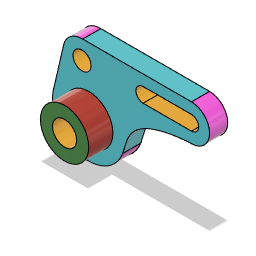
Questão4 (Autodesk Fusion 360 design; units mm, degrees)
Autodesk Fusion 360 part; units mm, degrees
sketch "Esboço1" plane through (0, 0, 0) normal (0, 0, 1) x (1, 0, 0)
  circle A0 centre (-75.5675, 24.3524) radius 7.5
  line L0 (-74.9976, 40) -> (15, 40)
  circle A1 centre (-70, -15) radius 10
  circle A2 centre (-70, -15) radius 20
  arc A3 (-74.9976, 40) -> (-91, 27) centre (-75.5675, 24.3524) ccw
  arc A4 (-98.6911, -6.2353) -> (-41.8777, -25.4469) centre (-70, -15) ccw
  line L1 (-91, 27) -> (-99.6247, -10.2696)
  spline S0 degree 5 poles (-41.8778, -25.447) (-41.2361, -23.7197) (-40.218, -20.1667) (-38.9242, -14.7529) (-36.1051, -8.0005) (-29.38, -1.1445) (-19.8049, 3.8654) (-8.8022, 7.1289) (1.7346, 8.9607) (9.9399, 9.7778) (14.6205, 10.0067) (15.4365, 10.0101) (15.3811, 10.0081) (15.4839, 10.0094) (15.5681, 10.0108) knots 0 0 0 0 0 0 0.1 0.2 0.3 0.4 0.5 0.6 0.7 0.8 0.9 1 1 1 1 1 1
  line L2 (7.592, 9.8796) -> (23.5441, 10.1419)
  arc A5 (15, 10) -> (15, 40) centre (15, 25) ccw
  line L3 (-25, 19) -> (15, 19)
  line L4 (15, 31) -> (-25, 31)
  arc A6 (-25, 31) -> (-25, 19) centre (-25, 25) ccw
  arc A7 (15, 19) -> (15, 31) centre (15, 25) ccw
  dimension "d3" = 12
  constraint concentric A0 A3
  constraint concentric A1 A2
  constraint concentric A2 A4
  constraint coincident A4 L1.end
  constraint coincident L1 A4.start
  constraint coincident A4 S0.start
  constraint midpoint S0.end L2
  constraint coincident S0 A4.end
  constraint tangent L3 A7
  measures "d3" diameter of A6
extrude "Extrusão1" add sketch "Esboço1" along normal blind 15 contours L0 A3 A4 L1 S0 L2 A5
sketch "Esboço2" plane through (0, 0, 0) normal (0, 0, -1) x (-1, 0, 0)
  circle A0 centre (75.5675, 24.3524) radius 7.5
  arc A1 (-15, 31) -> (-15, 19) centre (-15, 25) ccw
  line L0 (-15, 31) -> (25, 31)
  arc A2 (25, 19) -> (25, 31) centre (25, 25) ccw
  line L1 (25, 19) -> (-15, 19)
  circle A3 centre (70, -15) radius 20
  arc A4 (91, 27) -> (74.9976, 40) centre (75.5675, 24.3524) ccw
  line L2 (74.9976, 40) -> (-15, 40)
  arc A5 (-15, 40) -> (-15.5681, 10.0108) centre (-15, 25) ccw
  spline S0 degree 5 poles (41.8777, -25.4469) (41.2361, -23.7197) (40.218, -20.1666) (38.9242, -14.7529) (36.1051, -8.0004) (29.38, -1.1445) (19.8049, 3.8654) (8.8022, 7.1289) (-1.7346, 8.9607) (-9.9399, 9.7778) (-14.6205, 10.0067) (-15.4365, 10.0101) (-15.3811, 10.0081) (-15.4839, 10.0094) (-15.5681, 10.0108) knots 0.000001 0.000001 0.000001 0.000001 0.000001 0.000001 0.1 0.2 0.3 0.4 0.5 0.6 0.7 0.8 0.9 1 1 1 1 1 1
  line L3 (41.8777, -25.4469) -> (41.8778, -25.447)
  arc A6 (41.8778, -25.447) -> (99.6247, -10.2696) centre (70, -15) ccw
  line L4 (99.6247, -10.2696) -> (91, 27)
  circle A7 centre (70, -15) radius 20
  circle A8 centre (70, -15) radius 10
  dimension "d15" = 40
  dimension "d16" = 20
  constraint concentric A3 A7
  constraint concentric A7 A8
  measures "d15" diameter of A7
  measures "d16" diameter of A8
extrude "Extrusão2" add sketch "Esboço2" against normal blind 35 contours A3 A7
